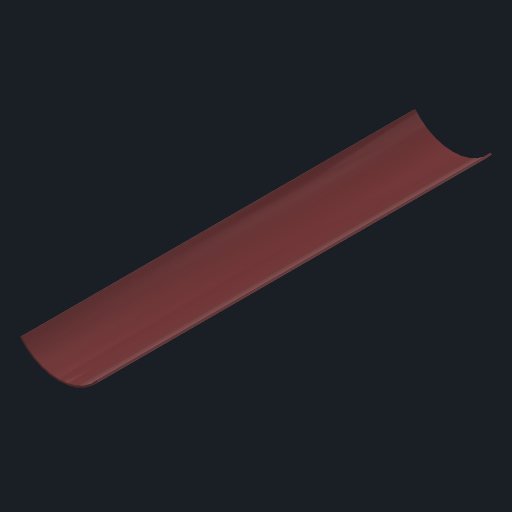
# Autodesk Inventor part: CANALETA_MOVIL
Saved by Autodesk Inventor 2024.3 (Build 283343000, 343)
## iProperties
Created: 2024-07-24
Part Number: CANALETA_MOVIL
Material: Steel, Mild, Welded
Document SubType Name: Modeling
Designer: Niler
Density: 7.85 g/cm^3
Appearance: Weld - Steel Mild
Author: Niler
Autodesk Inventor part; units mm, degrees
ref_plane "YZ Plane" through (0, 0, 0) normal (1, 0, 0) x (0, 1, 0)
ref_plane "XZ Plane" through (0, 0, 0) normal (0, 1, 0) x (-1, 0, 0)
ref_plane "XY Plane" through (0, 0, 0) normal (0, 0, 1) x (1, 0, 0)
sketch "Sketch1" plane through (0, 0, 0) normal (0, 0, 1) x (1, 0, 0)
  circle A0 centre (0, 0) radius 57.5
  circle A1 centre (0, 0) radius 59.5
  line L0 (0, 0) -> (-46.5, -37.1214)
  line L1 (0, 0) -> (0, 20.5864)
  line L2 (0, 0) -> (46.5, -37.1214)
  point P0 (46.5, -37.1214)
  point P1 (44.937, -35.8736)
  point P2 (-44.937, -35.8736)
  dimension "d0" = 115
  dimension "d1" = 2
  dimension "d2" = 93
  constraints: 6 end point, 1 centre point, 1 coincident, 1 symmetric about line, 1 vertical, 3 other
  measures "d0" diameter of A0
  measures "d2" distance of L2.end L0.end
extrude "Extrusion1" add sketch "Sketch1" along normal mid plane 470 contours A0 L2 A1 L0 picked at (-3.5394, -58.515)
body "Solid1"
